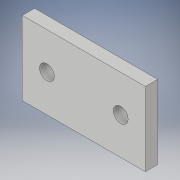
# Autodesk Inventor part: RelicArmSpacer
Saved by Autodesk Inventor 2017 (Build 210142000, 142)
## iProperties
Created: 2018-02-16
Part Number: RelicArmSpacer
Material: Generic
Document SubType Name: Modeling
Designer: User
Density: 1 g/cm^3
Appearance: Default
Author: User
Autodesk Inventor part; units mm, degrees
ref_plane "YZ Plane" through (0, 0, 0) normal (1, 0, 0) x (0, 1, 0)
ref_plane "XZ Plane" through (0, 0, 0) normal (0, 1, 0) x (-1, 0, 0)
ref_plane "XY Plane" through (0, 0, 0) normal (0, 0, 1) x (1, 0, 0)
sketch "Sketch1" plane through (0, 0, 0) normal (0, 0, 1) x (1, 0, 0)
  line L0 (0, 0) -> (63.5, 0)
  line L1 (63.5, 0) -> (63.5, 38.1)
  line L2 (63.5, 38.1) -> (0, 38.1)
  line L3 (0, 38.1) -> (0, 0)
  dimension "d0" = 63.5
  dimension "d1" = 38.1
  constraints: 8 end point, 2 parallel, 1 horizontal, 1 perpendicular
  measures "d0" distance of L2.end L1.end
  measures "d1" distance of L1.end L0.end
extrude "Extrusion1" add sketch "Sketch1" along normal blind 6.35
sketch "Sketch2" plane through (0, 0, 6.35) normal (0, 0, 1) x (1, 0, 0)
  line L0 (0, 38.1) -> (0, 0) projected
  line L1 (0, 19.05) -> (12.7, 19.05)
  line L2 (63.5, 0) -> (63.5, 38.1) projected
  line L3 (63.5, 19.05) -> (50.8, 19.05)
  line L4 (63.5, 19.05) -> (76.2, 19.05) construction
  dimension "d4" = 12.7
  dimension "d5" = 12.7
  dimension "d6" = 180
  constraints: 6 end point, 3 horizontal, 2 coincident, 2 midpoint, 1 collinear
  measures "d4" distance of L1.start L1.end
  measures "d5" distance of L3.start L3.end
  measures "d6" angle of L3 L4
hole "Hole1" at (12.7, 19.05, 6.35) at (50.8, 19.05, 6.35) direction (0, 0, -1) diameter 7.62 depth 25.4 tip angle 118
body "Solid1"
